Infidex176V-IDENTIDEM.design-remix-counter-train (Autodesk Fusion 360 design; units mm, degrees)
part number: 2026-09-16-11-02-38-314
part number: 2026-09-22-22-56-15-265
part number: 2026-09-22-22-56-15-756
part number: 2026-09-22-22-56-18-900
part number: 2026-09-22-22-56-23-574
part number: 2026-09-22-22-56-29-751
Autodesk Fusion 360 part; units mm, degrees
(part 1 of 7)
ref_plane "WorkPlane1" through (0, 0, 36.8) normal (0, 0, 1) x (1, 0, 0) in component "CT sprocket pinion (tool body)"
sketch "Sketch1" plane through (0, 0, 36.8) normal (0, 0, 1) x (1, 0, 0) in component "CT sprocket pinion (tool body)"
  line L0 (76.2524, -45.6906) -> (76.5417, -45.7362)
  line L1 (76.5417, -45.7362) -> (76.6223, -45.737)
  line L2 (76.6223, -45.737) -> (76.7043, -45.7279)
  line L3 (76.7043, -45.7279) -> (76.7872, -45.7118)
  line L4 (76.7872, -45.7118) -> (76.8707, -45.6898)
  line L5 (76.8707, -45.6898) -> (76.9545, -45.6623)
  line L6 (76.9545, -45.6623) -> (77.0386, -45.6298)
  line L7 (77.0386, -45.6298) -> (77.1226, -45.5924)
  line L8 (77.1226, -45.5924) -> (77.2065, -45.5504)
  line L9 (77.2065, -45.5504) -> (77.2902, -45.5039)
  line L10 (77.2902, -45.5039) -> (77.3734, -45.4529)
  line L11 (77.3734, -45.4529) -> (77.4561, -45.3975)
  line L12 (77.4561, -45.3975) -> (77.5381, -45.3379)
  line L13 (77.5381, -45.3379) -> (77.5398, -45.2526)
  line L14 (77.5398, -45.2526) -> (77.5398, -45.1674)
  line L15 (77.5398, -45.1674) -> (77.5381, -45.0821)
  line L16 (77.5381, -45.0821) -> (77.4561, -45.0225)
  line L17 (77.4561, -45.0225) -> (77.3734, -44.9671)
  line L18 (77.3734, -44.9671) -> (77.2902, -44.9161)
  line L19 (77.2902, -44.9161) -> (77.2065, -44.8696)
  line L20 (77.2065, -44.8696) -> (77.1226, -44.8276)
  line L21 (77.1226, -44.8276) -> (77.0386, -44.7902)
  line L22 (77.0386, -44.7902) -> (76.9545, -44.7577)
  line L23 (76.9545, -44.7577) -> (76.8707, -44.7302)
  line L24 (76.8707, -44.7302) -> (76.7872, -44.7082)
  line L25 (76.7872, -44.7082) -> (76.7043, -44.6921)
  line L26 (76.7043, -44.6921) -> (76.6223, -44.683)
  line L27 (76.6223, -44.683) -> (76.5417, -44.6838)
  line L28 (76.5417, -44.6838) -> (76.2524, -44.7294)
  line L29 (76.2524, -44.7294) -> (76.2228, -44.5689)
  line L30 (76.2228, -44.5689) -> (76.1847, -44.4102)
  line L31 (76.1847, -44.4102) -> (76.1383, -44.2538)
  line L32 (76.1383, -44.2538) -> (76.0838, -44.1)
  line L33 (76.0838, -44.1) -> (76.3571, -43.9948)
  line L34 (76.3571, -43.9948) -> (76.4273, -43.9553)
  line L35 (76.4273, -43.9553) -> (76.4938, -43.9063)
  line L36 (76.4938, -43.9063) -> (76.5575, -43.851)
  line L37 (76.5575, -43.851) -> (76.6188, -43.7901)
  line L38 (76.6188, -43.7901) -> (76.6777, -43.7244)
  line L39 (76.6777, -43.7244) -> (76.7342, -43.6543)
  line L40 (76.7342, -43.6543) -> (76.7883, -43.5799)
  line L41 (76.7883, -43.5799) -> (76.84, -43.5016)
  line L42 (76.84, -43.5016) -> (76.8891, -43.4194)
  line L43 (76.8891, -43.4194) -> (76.9357, -43.3336)
  line L44 (76.9357, -43.3336) -> (76.9797, -43.2444)
  line L45 (76.9797, -43.2444) -> (77.0209, -43.1517)
  line L46 (77.0209, -43.1517) -> (76.9797, -43.077)
  line L47 (76.9797, -43.077) -> (76.937, -43.0032)
  line L48 (76.937, -43.0032) -> (76.893, -42.9302)
  line L49 (76.893, -42.9302) -> (76.7921, -42.9195)
  line L50 (76.7921, -42.9195) -> (76.6929, -42.913)
  line L51 (76.6929, -42.913) -> (76.5953, -42.9104)
  line L52 (76.5953, -42.9104) -> (76.4995, -42.9119)
  line L53 (76.4995, -42.9119) -> (76.4059, -42.9175)
  line L54 (76.4059, -42.9175) -> (76.3144, -42.9272)
  line L55 (76.3144, -42.9272) -> (76.2254, -42.941)
  line L56 (76.2254, -42.941) -> (76.139, -42.9592)
  line L57 (76.139, -42.9592) -> (76.0557, -42.9818)
  line L58 (76.0557, -42.9818) -> (75.9759, -43.0093)
  line L59 (75.9759, -43.0093) -> (75.9003, -43.0424)
  line L60 (75.9003, -43.0424) -> (75.8309, -43.0834)
  line L61 (75.8309, -43.0834) -> (75.6031, -43.2676)
  line L62 (75.6031, -43.2676) -> (75.4972, -43.1434)
  line L63 (75.4972, -43.1434) -> (75.385, -43.025)
  line L64 (75.385, -43.025) -> (75.2666, -42.9128)
  line L65 (75.2666, -42.9128) -> (75.1424, -42.8069)
  line L66 (75.1424, -42.8069) -> (75.3266, -42.5791)
  line L67 (75.3266, -42.5791) -> (75.3676, -42.5097)
  line L68 (75.3676, -42.5097) -> (75.4007, -42.4341)
  line L69 (75.4007, -42.4341) -> (75.4282, -42.3543)
  line L70 (75.4282, -42.3543) -> (75.4508, -42.271)
  line L71 (75.4508, -42.271) -> (75.469, -42.1846)
  line L72 (75.469, -42.1846) -> (75.4828, -42.0956)
  line L73 (75.4828, -42.0956) -> (75.4925, -42.0041)
  line L74 (75.4925, -42.0041) -> (75.4981, -41.9105)
  line L75 (75.4981, -41.9105) -> (75.4996, -41.8147)
  line L76 (75.4996, -41.8147) -> (75.497, -41.7171)
  line L77 (75.497, -41.7171) -> (75.4905, -41.6179)
  line L78 (75.4905, -41.6179) -> (75.4798, -41.517)
  line L79 (75.4798, -41.517) -> (75.4068, -41.473)
  line L80 (75.4068, -41.473) -> (75.333, -41.4303)
  line L81 (75.333, -41.4303) -> (75.2583, -41.3891)
  line L82 (75.2583, -41.3891) -> (75.1656, -41.4303)
  line L83 (75.1656, -41.4303) -> (75.0764, -41.4743)
  line L84 (75.0764, -41.4743) -> (74.9906, -41.5209)
  line L85 (74.9906, -41.5209) -> (74.9084, -41.57)
  line L86 (74.9084, -41.57) -> (74.8301, -41.6217)
  line L87 (74.8301, -41.6217) -> (74.7557, -41.6758)
  line L88 (74.7557, -41.6758) -> (74.6856, -41.7323)
  line L89 (74.6856, -41.7323) -> (74.6199, -41.7912)
  line L90 (74.6199, -41.7912) -> (74.559, -41.8525)
  line L91 (74.559, -41.8525) -> (74.5037, -41.9162)
  line L92 (74.5037, -41.9162) -> (74.4547, -41.9827)
  line L93 (74.4547, -41.9827) -> (74.4152, -42.0529)
  line L94 (74.4152, -42.0529) -> (74.31, -42.3262)
  line L95 (74.31, -42.3262) -> (74.1562, -42.2717)
  line L96 (74.1562, -42.2717) -> (73.9998, -42.2253)
  line L97 (73.9998, -42.2253) -> (73.8411, -42.1872)
  line L98 (73.8411, -42.1872) -> (73.6806, -42.1576)
  line L99 (73.6806, -42.1576) -> (73.7262, -41.8683)
  line L100 (73.7262, -41.8683) -> (73.727, -41.7877)
  line L101 (73.727, -41.7877) -> (73.7179, -41.7057)
  line L102 (73.7179, -41.7057) -> (73.7018, -41.6228)
  line L103 (73.7018, -41.6228) -> (73.6798, -41.5393)
  line L104 (73.6798, -41.5393) -> (73.6523, -41.4555)
  line L105 (73.6523, -41.4555) -> (73.6198, -41.3714)
  line L106 (73.6198, -41.3714) -> (73.5824, -41.2874)
  line L107 (73.5824, -41.2874) -> (73.5404, -41.2035)
  line L108 (73.5404, -41.2035) -> (73.4939, -41.1198)
  line L109 (73.4939, -41.1198) -> (73.4429, -41.0366)
  line L110 (73.4429, -41.0366) -> (73.3875, -40.9539)
  line L111 (73.3875, -40.9539) -> (73.3279, -40.8719)
  line L112 (73.3279, -40.8719) -> (73.2426, -40.8702)
  line L113 (73.2426, -40.8702) -> (73.1574, -40.8702)
  line L114 (73.1574, -40.8702) -> (73.0721, -40.8719)
  line L115 (73.0721, -40.8719) -> (73.0125, -40.9539)
  line L116 (73.0125, -40.9539) -> (72.9571, -41.0366)
  line L117 (72.9571, -41.0366) -> (72.9061, -41.1198)
  line L118 (72.9061, -41.1198) -> (72.8596, -41.2035)
  line L119 (72.8596, -41.2035) -> (72.8176, -41.2874)
  line L120 (72.8176, -41.2874) -> (72.7802, -41.3714)
  line L121 (72.7802, -41.3714) -> (72.7477, -41.4555)
  line L122 (72.7477, -41.4555) -> (72.7202, -41.5393)
  line L123 (72.7202, -41.5393) -> (72.6982, -41.6228)
  line L124 (72.6982, -41.6228) -> (72.6821, -41.7057)
  line L125 (72.6821, -41.7057) -> (72.673, -41.7877)
  line L126 (72.673, -41.7877) -> (72.6738, -41.8683)
  line L127 (72.6738, -41.8683) -> (72.7194, -42.1576)
  line L128 (72.7194, -42.1576) -> (72.5589, -42.1872)
  line L129 (72.5589, -42.1872) -> (72.4002, -42.2253)
  line L130 (72.4002, -42.2253) -> (72.2438, -42.2717)
  line L131 (72.2438, -42.2717) -> (72.09, -42.3262)
  line L132 (72.09, -42.3262) -> (71.9848, -42.0529)
  line L133 (71.9848, -42.0529) -> (71.9453, -41.9827)
  line L134 (71.9453, -41.9827) -> (71.8963, -41.9162)
  line L135 (71.8963, -41.9162) -> (71.841, -41.8525)
  line L136 (71.841, -41.8525) -> (71.7801, -41.7912)
  line L137 (71.7801, -41.7912) -> (71.7144, -41.7323)
  line L138 (71.7144, -41.7323) -> (71.6443, -41.6758)
  line L139 (71.6443, -41.6758) -> (71.5699, -41.6217)
  line L140 (71.5699, -41.6217) -> (71.4916, -41.57)
  line L141 (71.4916, -41.57) -> (71.4094, -41.5209)
  line L142 (71.4094, -41.5209) -> (71.3236, -41.4743)
  line L143 (71.3236, -41.4743) -> (71.2344, -41.4303)
  line L144 (71.2344, -41.4303) -> (71.1417, -41.3891)
  line L145 (71.1417, -41.3891) -> (71.067, -41.4303)
  line L146 (71.067, -41.4303) -> (70.9932, -41.473)
  line L147 (70.9932, -41.473) -> (70.9202, -41.517)
  line L148 (70.9202, -41.517) -> (70.9095, -41.6179)
  line L149 (70.9095, -41.6179) -> (70.903, -41.7171)
  line L150 (70.903, -41.7171) -> (70.9004, -41.8147)
  line L151 (70.9004, -41.8147) -> (70.9019, -41.9105)
  line L152 (70.9019, -41.9105) -> (70.9075, -42.0041)
  line L153 (70.9075, -42.0041) -> (70.9172, -42.0956)
  line L154 (70.9172, -42.0956) -> (70.931, -42.1846)
  line L155 (70.931, -42.1846) -> (70.9492, -42.271)
  line L156 (70.9492, -42.271) -> (70.9718, -42.3543)
  line L157 (70.9718, -42.3543) -> (70.9993, -42.4341)
  line L158 (70.9993, -42.4341) -> (71.0324, -42.5097)
  line L159 (71.0324, -42.5097) -> (71.0734, -42.5791)
  line L160 (71.0734, -42.5791) -> (71.2576, -42.8069)
  line L161 (71.2576, -42.8069) -> (71.1334, -42.9128)
  line L162 (71.1334, -42.9128) -> (71.015, -43.025)
  line L163 (71.015, -43.025) -> (70.9028, -43.1434)
  line L164 (70.9028, -43.1434) -> (70.7969, -43.2676)
  line L165 (70.7969, -43.2676) -> (70.5691, -43.0834)
  line L166 (70.5691, -43.0834) -> (70.4997, -43.0424)
  line L167 (70.4997, -43.0424) -> (70.4241, -43.0093)
  line L168 (70.4241, -43.0093) -> (70.3443, -42.9818)
  line L169 (70.3443, -42.9818) -> (70.261, -42.9592)
  line L170 (70.261, -42.9592) -> (70.1746, -42.941)
  line L171 (70.1746, -42.941) -> (70.0856, -42.9272)
  line L172 (70.0856, -42.9272) -> (69.9941, -42.9175)
  line L173 (69.9941, -42.9175) -> (69.9005, -42.9119)
  line L174 (69.9005, -42.9119) -> (69.8047, -42.9104)
  line L175 (69.8047, -42.9104) -> (69.7071, -42.913)
  line L176 (69.7071, -42.913) -> (69.6079, -42.9195)
  line L177 (69.6079, -42.9195) -> (69.507, -42.9302)
  line L178 (69.507, -42.9302) -> (69.463, -43.0032)
  line L179 (69.463, -43.0032) -> (69.4203, -43.077)
  line L180 (69.4203, -43.077) -> (69.3791, -43.1517)
  line L181 (69.3791, -43.1517) -> (69.4203, -43.2444)
  line L182 (69.4203, -43.2444) -> (69.4643, -43.3336)
  line L183 (69.4643, -43.3336) -> (69.5109, -43.4194)
  line L184 (69.5109, -43.4194) -> (69.56, -43.5016)
  line L185 (69.56, -43.5016) -> (69.6117, -43.5799)
  line L186 (69.6117, -43.5799) -> (69.6658, -43.6543)
  line L187 (69.6658, -43.6543) -> (69.7223, -43.7244)
  line L188 (69.7223, -43.7244) -> (69.7812, -43.7901)
  line L189 (69.7812, -43.7901) -> (69.8425, -43.851)
  line L190 (69.8425, -43.851) -> (69.9062, -43.9063)
  line L191 (69.9062, -43.9063) -> (69.9727, -43.9553)
  line L192 (69.9727, -43.9553) -> (70.0429, -43.9948)
  line L193 (70.0429, -43.9948) -> (70.3162, -44.1)
  line L194 (70.3162, -44.1) -> (70.2617, -44.2538)
  line L195 (70.2617, -44.2538) -> (70.2153, -44.4102)
  line L196 (70.2153, -44.4102) -> (70.1772, -44.5689)
  line L197 (70.1772, -44.5689) -> (70.1476, -44.7294)
  line L198 (70.1476, -44.7294) -> (69.8583, -44.6838)
  line L199 (69.8583, -44.6838) -> (69.7777, -44.683)
  line L200 (69.7777, -44.683) -> (69.6957, -44.6921)
  line L201 (69.6957, -44.6921) -> (69.6128, -44.7082)
  line L202 (69.6128, -44.7082) -> (69.5293, -44.7302)
  line L203 (69.5293, -44.7302) -> (69.4455, -44.7577)
  line L204 (69.4455, -44.7577) -> (69.3614, -44.7902)
  line L205 (69.3614, -44.7902) -> (69.2774, -44.8276)
  line L206 (69.2774, -44.8276) -> (69.1935, -44.8696)
  line L207 (69.1935, -44.8696) -> (69.1098, -44.9161)
  line L208 (69.1098, -44.9161) -> (69.0266, -44.9671)
  line L209 (69.0266, -44.9671) -> (68.9439, -45.0225)
  line L210 (68.9439, -45.0225) -> (68.8619, -45.0821)
  line L211 (68.8619, -45.0821) -> (68.8602, -45.1674)
  line L212 (68.8602, -45.1674) -> (68.8602, -45.2526)
  line L213 (68.8602, -45.2526) -> (68.8619, -45.3379)
  line L214 (68.8619, -45.3379) -> (68.9439, -45.3975)
  line L215 (68.9439, -45.3975) -> (69.0266, -45.4529)
  line L216 (69.0266, -45.4529) -> (69.1098, -45.5039)
  line L217 (69.1098, -45.5039) -> (69.1935, -45.5504)
  line L218 (69.1935, -45.5504) -> (69.2774, -45.5924)
  line L219 (69.2774, -45.5924) -> (69.3614, -45.6298)
  line L220 (69.3614, -45.6298) -> (69.4455, -45.6623)
  line L221 (69.4455, -45.6623) -> (69.5293, -45.6898)
  line L222 (69.5293, -45.6898) -> (69.6128, -45.7118)
  line L223 (69.6128, -45.7118) -> (69.6957, -45.7279)
  line L224 (69.6957, -45.7279) -> (69.7777, -45.737)
  line L225 (69.7777, -45.737) -> (69.8583, -45.7362)
  line L226 (69.8583, -45.7362) -> (70.1476, -45.6906)
  line L227 (70.1476, -45.6906) -> (70.1772, -45.8511)
  line L228 (70.1772, -45.8511) -> (70.2153, -46.0098)
  line L229 (70.2153, -46.0098) -> (70.2617, -46.1662)
  line L230 (70.2617, -46.1662) -> (70.3162, -46.32)
  line L231 (70.3162, -46.32) -> (70.0429, -46.4252)
  line L232 (70.0429, -46.4252) -> (69.9727, -46.4647)
  line L233 (69.9727, -46.4647) -> (69.9062, -46.5137)
  line L234 (69.9062, -46.5137) -> (69.8425, -46.569)
  line L235 (69.8425, -46.569) -> (69.7812, -46.6299)
  line L236 (69.7812, -46.6299) -> (69.7223, -46.6956)
  line L237 (69.7223, -46.6956) -> (69.6658, -46.7657)
  line L238 (69.6658, -46.7657) -> (69.6117, -46.8401)
  line L239 (69.6117, -46.8401) -> (69.56, -46.9184)
  line L240 (69.56, -46.9184) -> (69.5109, -47.0006)
  line L241 (69.5109, -47.0006) -> (69.4643, -47.0864)
  line L242 (69.4643, -47.0864) -> (69.4203, -47.1756)
  line L243 (69.4203, -47.1756) -> (69.3791, -47.2683)
  line L244 (69.3791, -47.2683) -> (69.4203, -47.343)
  line L245 (69.4203, -47.343) -> (69.463, -47.4168)
  line L246 (69.463, -47.4168) -> (69.507, -47.4898)
  line L247 (69.507, -47.4898) -> (69.6079, -47.5005)
  line L248 (69.6079, -47.5005) -> (69.7071, -47.507)
  line L249 (69.7071, -47.507) -> (69.8047, -47.5096)
  line L250 (69.8047, -47.5096) -> (69.9005, -47.5081)
  line L251 (69.9005, -47.5081) -> (69.9941, -47.5025)
  line L252 (69.9941, -47.5025) -> (70.0856, -47.4928)
  line L253 (70.0856, -47.4928) -> (70.1746, -47.479)
  line L254 (70.1746, -47.479) -> (70.261, -47.4608)
  line L255 (70.261, -47.4608) -> (70.3443, -47.4382)
  line L256 (70.3443, -47.4382) -> (70.4241, -47.4107)
  line L257 (70.4241, -47.4107) -> (70.4997, -47.3776)
  line L258 (70.4997, -47.3776) -> (70.5691, -47.3366)
  line L259 (70.5691, -47.3366) -> (70.7969, -47.1524)
  line L260 (70.7969, -47.1524) -> (70.9028, -47.2766)
  line L261 (70.9028, -47.2766) -> (71.015, -47.395)
  line L262 (71.015, -47.395) -> (71.1334, -47.5072)
  line L263 (71.1334, -47.5072) -> (71.2576, -47.6131)
  line L264 (71.2576, -47.6131) -> (71.0734, -47.8409)
  line L265 (71.0734, -47.8409) -> (71.0324, -47.9103)
  line L266 (71.0324, -47.9103) -> (70.9993, -47.9859)
  line L267 (70.9993, -47.9859) -> (70.9718, -48.0657)
  line L268 (70.9718, -48.0657) -> (70.9492, -48.149)
  line L269 (70.9492, -48.149) -> (70.931, -48.2354)
  line L270 (70.931, -48.2354) -> (70.9172, -48.3244)
  line L271 (70.9172, -48.3244) -> (70.9075, -48.4159)
  line L272 (70.9075, -48.4159) -> (70.9019, -48.5095)
  line L273 (70.9019, -48.5095) -> (70.9004, -48.6053)
  line L274 (70.9004, -48.6053) -> (70.903, -48.7029)
  line L275 (70.903, -48.7029) -> (70.9095, -48.8021)
  line L276 (70.9095, -48.8021) -> (70.9202, -48.903)
  line L277 (70.9202, -48.903) -> (70.9932, -48.947)
  line L278 (70.9932, -48.947) -> (71.067, -48.9897)
  line L279 (71.067, -48.9897) -> (71.1417, -49.0309)
  line L280 (71.1417, -49.0309) -> (71.2344, -48.9897)
  line L281 (71.2344, -48.9897) -> (71.3236, -48.9457)
  line L282 (71.3236, -48.9457) -> (71.4094, -48.8991)
  line L283 (71.4094, -48.8991) -> (71.4916, -48.85)
  line L284 (71.4916, -48.85) -> (71.5699, -48.7983)
  line L285 (71.5699, -48.7983) -> (71.6443, -48.7442)
  line L286 (71.6443, -48.7442) -> (71.7144, -48.6877)
  line L287 (71.7144, -48.6877) -> (71.7801, -48.6288)
  line L288 (71.7801, -48.6288) -> (71.841, -48.5675)
  line L289 (71.841, -48.5675) -> (71.8963, -48.5038)
  line L290 (71.8963, -48.5038) -> (71.9453, -48.4373)
  line L291 (71.9453, -48.4373) -> (71.9848, -48.3671)
  line L292 (71.9848, -48.3671) -> (72.09, -48.0938)
  line L293 (72.09, -48.0938) -> (72.2438, -48.1483)
  line L294 (72.2438, -48.1483) -> (72.4002, -48.1947)
  line L295 (72.4002, -48.1947) -> (72.5589, -48.2328)
  line L296 (72.5589, -48.2328) -> (72.7194, -48.2624)
  line L297 (72.7194, -48.2624) -> (72.6738, -48.5517)
  line L298 (72.6738, -48.5517) -> (72.673, -48.6323)
  line L299 (72.673, -48.6323) -> (72.6821, -48.7143)
  line L300 (72.6821, -48.7143) -> (72.6982, -48.7972)
  line L301 (72.6982, -48.7972) -> (72.7202, -48.8807)
  line L302 (72.7202, -48.8807) -> (72.7477, -48.9645)
  line L303 (72.7477, -48.9645) -> (72.7802, -49.0486)
  line L304 (72.7802, -49.0486) -> (72.8176, -49.1326)
  line L305 (72.8176, -49.1326) -> (72.8596, -49.2165)
  line L306 (72.8596, -49.2165) -> (72.9061, -49.3002)
  line L307 (72.9061, -49.3002) -> (72.9571, -49.3834)
  line L308 (72.9571, -49.3834) -> (73.0125, -49.4661)
  line L309 (73.0125, -49.4661) -> (73.0721, -49.5481)
  line L310 (73.0721, -49.5481) -> (73.1574, -49.5498)
  line L311 (73.1574, -49.5498) -> (73.2426, -49.5498)
  line L312 (73.2426, -49.5498) -> (73.3279, -49.5481)
  line L313 (73.3279, -49.5481) -> (73.3875, -49.4661)
  line L314 (73.3875, -49.4661) -> (73.4429, -49.3834)
  line L315 (73.4429, -49.3834) -> (73.4939, -49.3002)
  line L316 (73.4939, -49.3002) -> (73.5404, -49.2165)
  line L317 (73.5404, -49.2165) -> (73.5824, -49.1326)
  line L318 (73.5824, -49.1326) -> (73.6198, -49.0486)
  line L319 (73.6198, -49.0486) -> (73.6523, -48.9645)
  line L320 (73.6523, -48.9645) -> (73.6798, -48.8807)
  line L321 (73.6798, -48.8807) -> (73.7018, -48.7972)
  line L322 (73.7018, -48.7972) -> (73.7179, -48.7143)
  line L323 (73.7179, -48.7143) -> (73.727, -48.6323)
  line L324 (73.727, -48.6323) -> (73.7262, -48.5517)
  line L325 (73.7262, -48.5517) -> (73.6806, -48.2624)
  line L326 (73.6806, -48.2624) -> (73.8411, -48.2328)
  line L327 (73.8411, -48.2328) -> (73.9998, -48.1947)
  line L328 (73.9998, -48.1947) -> (74.1562, -48.1483)
  line L329 (74.1562, -48.1483) -> (74.31, -48.0938)
  line L330 (74.31, -48.0938) -> (74.4152, -48.3671)
  line L331 (74.4152, -48.3671) -> (74.4547, -48.4373)
  line L332 (74.4547, -48.4373) -> (74.5037, -48.5038)
  line L333 (74.5037, -48.5038) -> (74.559, -48.5675)
  line L334 (74.559, -48.5675) -> (74.6199, -48.6288)
  line L335 (74.6199, -48.6288) -> (74.6856, -48.6877)
  line L336 (74.6856, -48.6877) -> (74.7557, -48.7442)
  line L337 (74.7557, -48.7442) -> (74.8301, -48.7983)
  line L338 (74.8301, -48.7983) -> (74.9084, -48.85)
  line L339 (74.9084, -48.85) -> (74.9906, -48.8991)
  line L340 (74.9906, -48.8991) -> (75.0764, -48.9457)
  line L341 (75.0764, -48.9457) -> (75.1656, -48.9897)
  line L342 (75.1656, -48.9897) -> (75.2583, -49.0309)
  line L343 (75.2583, -49.0309) -> (75.333, -48.9897)
  line L344 (75.333, -48.9897) -> (75.4068, -48.947)
  line L345 (75.4068, -48.947) -> (75.4798, -48.903)
  line L346 (75.4798, -48.903) -> (75.4905, -48.8021)
  line L347 (75.4905, -48.8021) -> (75.497, -48.7029)
  line L348 (75.497, -48.7029) -> (75.4996, -48.6053)
  line L349 (75.4996, -48.6053) -> (75.4981, -48.5095)
  line L350 (75.4981, -48.5095) -> (75.4925, -48.4159)
  line L351 (75.4925, -48.4159) -> (75.4828, -48.3244)
  line L352 (75.4828, -48.3244) -> (75.469, -48.2354)
  line L353 (75.469, -48.2354) -> (75.4508, -48.149)
  line L354 (75.4508, -48.149) -> (75.4282, -48.0657)
  line L355 (75.4282, -48.0657) -> (75.4007, -47.9859)
  line L356 (75.4007, -47.9859) -> (75.3676, -47.9103)
  line L357 (75.3676, -47.9103) -> (75.3266, -47.8409)
  line L358 (75.3266, -47.8409) -> (75.1424, -47.6131)
  line L359 (75.1424, -47.6131) -> (75.2666, -47.5072)
  line L360 (75.2666, -47.5072) -> (75.385, -47.395)
  line L361 (75.385, -47.395) -> (75.4972, -47.2766)
  line L362 (75.4972, -47.2766) -> (75.6031, -47.1524)
  line L363 (75.6031, -47.1524) -> (75.8309, -47.3366)
  line L364 (75.8309, -47.3366) -> (75.9003, -47.3776)
  line L365 (75.9003, -47.3776) -> (75.9759, -47.4107)
  line L366 (75.9759, -47.4107) -> (76.0557, -47.4382)
  line L367 (76.0557, -47.4382) -> (76.139, -47.4608)
  line L368 (76.139, -47.4608) -> (76.2254, -47.479)
  line L369 (76.2254, -47.479) -> (76.3144, -47.4928)
  line L370 (76.3144, -47.4928) -> (76.4059, -47.5025)
  line L371 (76.4059, -47.5025) -> (76.4995, -47.5081)
  line L372 (76.4995, -47.5081) -> (76.5953, -47.5096)
  line L373 (76.5953, -47.5096) -> (76.6929, -47.507)
  line L374 (76.6929, -47.507) -> (76.7921, -47.5005)
  line L375 (76.7921, -47.5005) -> (76.893, -47.4898)
  line L376 (76.893, -47.4898) -> (76.937, -47.4168)
  line L377 (76.937, -47.4168) -> (76.9797, -47.343)
  line L378 (76.9797, -47.343) -> (77.0209, -47.2683)
  line L379 (77.0209, -47.2683) -> (76.9797, -47.1756)
  line L380 (76.9797, -47.1756) -> (76.9357, -47.0864)
  line L381 (76.9357, -47.0864) -> (76.8891, -47.0006)
  line L382 (76.8891, -47.0006) -> (76.84, -46.9184)
  line L383 (76.84, -46.9184) -> (76.7883, -46.8401)
  line L384 (76.7883, -46.8401) -> (76.7342, -46.7657)
  line L385 (76.7342, -46.7657) -> (76.6777, -46.6956)
  line L386 (76.6777, -46.6956) -> (76.6188, -46.6299)
  line L387 (76.6188, -46.6299) -> (76.5575, -46.569)
  line L388 (76.5575, -46.569) -> (76.4938, -46.5137)
  line L389 (76.4938, -46.5137) -> (76.4273, -46.4647)
  line L390 (76.4273, -46.4647) -> (76.3571, -46.4252)
  line L391 (76.3571, -46.4252) -> (76.0838, -46.32)
  line L392 (76.0838, -46.32) -> (76.1383, -46.1662)
  line L393 (76.1383, -46.1662) -> (76.1847, -46.0098)
  line L394 (76.1847, -46.0098) -> (76.2228, -45.8511)
  line L395 (76.2228, -45.8511) -> (76.2524, -45.6906)
extrude "Extrude1" add sketch "Sketch1" along normal blind 2 makes body 1 in component "CT sprocket pinion (tool body)"
ref_plane "WorkPlane1" through (0, 0, 36.8) normal (0, 0, 1) x (1, 0, 0) in component "CT idler 1"
sketch "Sketch1 (2)" plane through (0, 0, 36.8) normal (0, 0, 1) x (1, 0, 0) in component "CT idler 1"
  line L0 (81.6289, -58.8365) -> (82.0394, -58.8569)
  line L1 (82.0394, -58.8569) -> (82.1146, -58.8542)
  line L2 (82.1146, -58.8542) -> (82.19, -58.846)
  line L3 (82.19, -58.846) -> (82.2655, -58.8342)
  line L4 (82.2655, -58.8342) -> (82.3412, -58.8194)
  line L5 (82.3412, -58.8194) -> (82.4169, -58.802)
  line L6 (82.4169, -58.802) -> (82.4927, -58.7822)
  line L7 (82.4927, -58.7822) -> (82.5685, -58.7601)
  line L8 (82.5685, -58.7601) -> (82.6443, -58.7359)
  line L9 (82.6443, -58.7359) -> (82.7201, -58.7098)
  line L10 (82.7201, -58.7098) -> (82.7959, -58.6817)
  line L11 (82.7959, -58.6817) -> (82.8716, -58.6517)
  line L12 (82.8716, -58.6517) -> (82.9473, -58.6199)
  line L13 (82.9473, -58.6199) -> (82.9493, -58.4792)
  line L14 (82.9493, -58.4792) -> (82.9493, -58.3386)
  line L15 (82.9493, -58.3386) -> (82.9473, -58.1979)
  line L16 (82.9473, -58.1979) -> (82.8716, -58.1661)
  line L17 (82.8716, -58.1661) -> (82.7959, -58.1361)
  line L18 (82.7959, -58.1361) -> (82.7201, -58.108)
  line L19 (82.7201, -58.108) -> (82.6443, -58.0818)
  line L20 (82.6443, -58.0818) -> (82.5685, -58.0577)
  line L21 (82.5685, -58.0577) -> (82.4927, -58.0356)
  line L22 (82.4927, -58.0356) -> (82.4169, -58.0158)
  line L23 (82.4169, -58.0158) -> (82.3412, -57.9984)
  line L24 (82.3412, -57.9984) -> (82.2655, -57.9836)
  line L25 (82.2655, -57.9836) -> (82.19, -57.9718)
  line L26 (82.19, -57.9718) -> (82.1146, -57.9636)
  line L27 (82.1146, -57.9636) -> (82.0394, -57.9609)
  line L28 (82.0394, -57.9609) -> (81.6289, -57.9813)
  line L29 (81.6289, -57.9813) -> (81.616, -57.7729)
  line L30 (81.616, -57.7729) -> (81.5981, -57.565)
  line L31 (81.5981, -57.565) -> (81.5751, -57.3575)
  line L32 (81.5751, -57.3575) -> (81.5471, -57.1506)
  line L33 (81.5471, -57.1506) -> (81.9537, -57.0906)
  line L34 (81.9537, -57.0906) -> (82.0269, -57.0732)
  line L35 (82.0269, -57.0732) -> (82.0992, -57.0505)
  line L36 (82.0992, -57.0505) -> (82.171, -57.0242)
  line L37 (82.171, -57.0242) -> (82.2423, -56.9949)
  line L38 (82.2423, -56.9949) -> (82.3132, -56.9631)
  line L39 (82.3132, -56.9631) -> (82.3837, -56.9288)
  line L40 (82.3837, -56.9288) -> (82.4537, -56.8924)
  line L41 (82.4537, -56.8924) -> (82.5234, -56.8539)
  line L42 (82.5234, -56.8539) -> (82.5926, -56.8134)
  line L43 (82.5926, -56.8134) -> (82.6614, -56.7711)
  line L44 (82.6614, -56.7711) -> (82.7299, -56.7269)
  line L45 (82.7299, -56.7269) -> (82.7979, -56.681)
  line L46 (82.7979, -56.681) -> (82.7724, -56.5426)
  line L47 (82.7724, -56.5426) -> (82.7449, -56.4047)
  line L48 (82.7449, -56.4047) -> (82.7155, -56.2671)
  line L49 (82.7155, -56.2671) -> (82.6351, -56.2507)
  line L50 (82.6351, -56.2507) -> (82.555, -56.2361)
  line L51 (82.555, -56.2361) -> (82.4752, -56.2233)
  line L52 (82.4752, -56.2233) -> (82.3958, -56.2124)
  line L53 (82.3958, -56.2124) -> (82.3167, -56.2035)
  line L54 (82.3167, -56.2035) -> (82.238, -56.1966)
  line L55 (82.238, -56.1966) -> (82.1598, -56.192)
  line L56 (82.1598, -56.192) -> (82.0822, -56.1896)
  line L57 (82.0822, -56.1896) -> (82.0051, -56.1899)
  line L58 (82.0051, -56.1899) -> (81.9287, -56.1931)
  line L59 (81.9287, -56.1931) -> (81.8531, -56.1998)
  line L60 (81.8531, -56.1998) -> (81.7789, -56.2117)
  line L61 (81.7789, -56.2117) -> (81.3802, -56.3119)
  line L62 (81.3802, -56.3119) -> (81.3269, -56.11)
  line L63 (81.3269, -56.11) -> (81.2688, -55.9095)
  line L64 (81.2688, -55.9095) -> (81.2058, -55.7105)
  line L65 (81.2058, -55.7105) -> (81.1379, -55.5131)
  line L66 (81.1379, -55.5131) -> (81.525, -55.3749)
  line L67 (81.525, -55.3749) -> (81.5934, -55.3436)
  line L68 (81.5934, -55.3436) -> (81.6599, -55.3072)
  line L69 (81.6599, -55.3072) -> (81.7252, -55.2674)
  line L70 (81.7252, -55.2674) -> (81.7895, -55.2248)
  line L71 (81.7895, -55.2248) -> (81.8528, -55.1797)
  line L72 (81.8528, -55.1797) -> (81.9152, -55.1324)
  line L73 (81.9152, -55.1324) -> (81.9768, -55.083)
  line L74 (81.9768, -55.083) -> (82.0376, -55.0316)
  line L75 (82.0376, -55.0316) -> (82.0976, -54.9784)
  line L76 (82.0976, -54.9784) -> (82.1568, -54.9235)
  line L77 (82.1568, -54.9235) -> (82.2153, -54.8668)
  line L78 (82.2153, -54.8668) -> (82.2731, -54.8085)
  line L79 (82.2731, -54.8085) -> (82.2211, -54.6778)
  line L80 (82.2211, -54.6778) -> (82.1673, -54.5478)
  line L81 (82.1673, -54.5478) -> (82.1116, -54.4186)
  line L82 (82.1116, -54.4186) -> (82.0295, -54.4182)
  line L83 (82.0295, -54.4182) -> (81.9481, -54.4195)
  line L84 (81.9481, -54.4195) -> (81.8673, -54.4225)
  line L85 (81.8673, -54.4225) -> (81.7873, -54.4273)
  line L86 (81.7873, -54.4273) -> (81.708, -54.434)
  line L87 (81.708, -54.434) -> (81.6295, -54.4426)
  line L88 (81.6295, -54.4426) -> (81.5519, -54.4533)
  line L89 (81.5519, -54.4533) -> (81.4753, -54.4662)
  line L90 (81.4753, -54.4662) -> (81.3997, -54.4815)
  line L91 (81.3997, -54.4815) -> (81.3254, -54.4995)
  line L92 (81.3254, -54.4995) -> (81.2526, -54.5208)
  line L93 (81.2526, -54.5208) -> (81.1821, -54.547)
  line L94 (81.1821, -54.547) -> (80.8107, -54.723)
  line L95 (80.8107, -54.723) -> (80.719, -54.5355)
  line L96 (80.719, -54.5355) -> (80.6229, -54.3502)
  line L97 (80.6229, -54.3502) -> (80.5222, -54.1673)
  line L98 (80.5222, -54.1673) -> (80.4172, -53.9869)
  line L99 (80.4172, -53.9869) -> (80.7699, -53.7758)
  line L100 (80.7699, -53.7758) -> (80.8309, -53.7318)
  line L101 (80.8309, -53.7318) -> (80.889, -53.6831)
  line L102 (80.889, -53.6831) -> (80.9453, -53.6313)
  line L103 (80.9453, -53.6313) -> (81, -53.577)
  line L104 (81, -53.577) -> (81.0532, -53.5204)
  line L105 (81.0532, -53.5204) -> (81.1052, -53.4618)
  line L106 (81.1052, -53.4618) -> (81.156, -53.4014)
  line L107 (81.156, -53.4014) -> (81.2056, -53.3391)
  line L108 (81.2056, -53.3391) -> (81.2541, -53.2753)
  line L109 (81.2541, -53.2753) -> (81.3015, -53.2098)
  line L110 (81.3015, -53.2098) -> (81.3478, -53.1428)
  line L111 (81.3478, -53.1428) -> (81.3931, -53.0743)
  line L112 (81.3931, -53.0743) -> (81.3166, -52.9563)
  line L113 (81.3166, -52.9563) -> (81.2384, -52.8393)
  line L114 (81.2384, -52.8393) -> (81.1586, -52.7234)
  line L115 (81.1586, -52.7234) -> (81.078, -52.7391)
  line L116 (81.078, -52.7391) -> (80.9984, -52.7562)
  line L117 (80.9984, -52.7562) -> (80.9198, -52.7749)
  line L118 (80.9198, -52.7749) -> (80.8422, -52.7953)
  line L119 (80.8422, -52.7953) -> (80.7658, -52.8173)
  line L120 (80.7658, -52.8173) -> (80.6905, -52.8411)
  line L121 (80.6905, -52.8411) -> (80.6164, -52.8667)
  line L122 (80.6164, -52.8667) -> (80.5438, -52.8943)
  line L123 (80.5438, -52.8943) -> (80.4727, -52.924)
  line L124 (80.4727, -52.924) -> (80.4033, -52.9562)
  line L125 (80.4033, -52.9562) -> (80.3361, -52.9913)
  line L126 (80.3361, -52.9913) -> (80.2721, -53.0307)
  line L127 (80.2721, -53.0307) -> (79.9421, -53.2758)
  line L128 (79.9421, -53.2758) -> (79.8156, -53.1097)
  line L129 (79.8156, -53.1097) -> (79.6851, -52.9468)
  line L130 (79.6851, -52.9468) -> (79.5508, -52.787)
  line L131 (79.5508, -52.787) -> (79.4126, -52.6306)
  line L132 (79.4126, -52.6306) -> (79.7173, -52.3547)
  line L133 (79.7173, -52.3547) -> (79.7685, -52.2997)
  line L134 (79.7685, -52.2997) -> (79.816, -52.2406)
  line L135 (79.816, -52.2406) -> (79.8611, -52.1788)
  line L136 (79.8611, -52.1788) -> (79.9041, -52.1149)
  line L137 (79.9041, -52.1149) -> (79.9454, -52.049)
  line L138 (79.9454, -52.049) -> (79.9849, -51.9814)
  line L139 (79.9849, -51.9814) -> (80.0229, -51.9122)
  line L140 (80.0229, -51.9122) -> (80.0595, -51.8415)
  line L141 (80.0595, -51.8415) -> (80.0945, -51.7694)
  line L142 (80.0945, -51.7694) -> (80.1283, -51.6959)
  line L143 (80.1283, -51.6959) -> (80.1606, -51.6212)
  line L144 (80.1606, -51.6212) -> (80.1916, -51.5452)
  line L145 (80.1916, -51.5452) -> (80.0936, -51.4443)
  line L146 (80.0936, -51.4443) -> (79.9941, -51.3448)
  line L147 (79.9941, -51.3448) -> (79.8932, -51.2468)
  line L148 (79.8932, -51.2468) -> (79.8173, -51.2778)
  line L149 (79.8173, -51.2778) -> (79.7425, -51.3102)
  line L150 (79.7425, -51.3102) -> (79.6691, -51.3439)
  line L151 (79.6691, -51.3439) -> (79.5969, -51.379)
  line L152 (79.5969, -51.379) -> (79.5262, -51.4155)
  line L153 (79.5262, -51.4155) -> (79.457, -51.4535)
  line L154 (79.457, -51.4535) -> (79.3894, -51.493)
  line L155 (79.3894, -51.493) -> (79.3236, -51.5343)
  line L156 (79.3236, -51.5343) -> (79.2596, -51.5773)
  line L157 (79.2596, -51.5773) -> (79.1979, -51.6224)
  line L158 (79.1979, -51.6224) -> (79.1388, -51.6699)
  line L159 (79.1388, -51.6699) -> (79.0837, -51.7211)
  line L160 (79.0837, -51.7211) -> (78.8078, -52.0259)
  line L161 (78.8078, -52.0259) -> (78.6514, -51.8877)
  line L162 (78.6514, -51.8877) -> (78.4916, -51.7533)
  line L163 (78.4916, -51.7533) -> (78.3287, -51.6228)
  line L164 (78.3287, -51.6228) -> (78.1626, -51.4963)
  line L165 (78.1626, -51.4963) -> (78.4077, -51.1663)
  line L166 (78.4077, -51.1663) -> (78.4471, -51.1023)
  line L167 (78.4471, -51.1023) -> (78.4822, -51.0351)
  line L168 (78.4822, -51.0351) -> (78.5144, -50.9657)
  line L169 (78.5144, -50.9657) -> (78.5441, -50.8946)
  line L170 (78.5441, -50.8946) -> (78.5717, -50.822)
  line L171 (78.5717, -50.822) -> (78.5974, -50.748)
  line L172 (78.5974, -50.748) -> (78.6211, -50.6727)
  line L173 (78.6211, -50.6727) -> (78.6431, -50.5962)
  line L174 (78.6431, -50.5962) -> (78.6635, -50.5186)
  line L175 (78.6635, -50.5186) -> (78.6822, -50.44)
  line L176 (78.6822, -50.44) -> (78.6994, -50.3604)
  line L177 (78.6994, -50.3604) -> (78.715, -50.2798)
  line L178 (78.715, -50.2798) -> (78.5991, -50.2)
  line L179 (78.5991, -50.2) -> (78.4822, -50.1219)
  line L180 (78.4822, -50.1219) -> (78.3641, -50.0454)
  line L181 (78.3641, -50.0454) -> (78.2956, -50.0906)
  line L182 (78.2956, -50.0906) -> (78.2286, -50.1369)
  line L183 (78.2286, -50.1369) -> (78.1632, -50.1843)
  line L184 (78.1632, -50.1843) -> (78.0993, -50.2328)
  line L185 (78.0993, -50.2328) -> (78.0371, -50.2824)
  line L186 (78.0371, -50.2824) -> (77.9766, -50.3332)
  line L187 (77.9766, -50.3332) -> (77.918, -50.3852)
  line L188 (77.918, -50.3852) -> (77.8615, -50.4385)
  line L189 (77.8615, -50.4385) -> (77.8071, -50.4932)
  line L190 (77.8071, -50.4932) -> (77.7553, -50.5494)
  line L191 (77.7553, -50.5494) -> (77.7067, -50.6076)
  line L192 (77.7067, -50.6076) -> (77.6626, -50.6685)
  line L193 (77.6626, -50.6685) -> (77.4515, -51.0212)
  line L194 (77.4515, -51.0212) -> (77.2711, -50.9162)
  line L195 (77.2711, -50.9162) -> (77.0882, -50.8156)
  line L196 (77.0882, -50.8156) -> (76.903, -50.7194)
  line L197 (76.903, -50.7194) -> (76.7154, -50.6277)
  line L198 (76.7154, -50.6277) -> (76.8914, -50.2563)
  line L199 (76.8914, -50.2563) -> (76.9176, -50.1858)
  line L200 (76.9176, -50.1858) -> (76.9389, -50.113)
  line L201 (76.9389, -50.113) -> (76.9569, -50.0387)
  line L202 (76.9569, -50.0387) -> (76.9722, -49.9632)
  line L203 (76.9722, -49.9632) -> (76.9851, -49.8865)
  line L204 (76.9851, -49.8865) -> (76.9958, -49.8089)
  line L205 (76.9958, -49.8089) -> (77.0044, -49.7304)
  line L206 (77.0044, -49.7304) -> (77.0111, -49.6511)
  line L207 (77.0111, -49.6511) -> (77.0159, -49.5711)
  line L208 (77.0159, -49.5711) -> (77.0189, -49.4903)
  line L209 (77.0189, -49.4903) -> (77.0202, -49.4089)
  line L210 (77.0202, -49.4089) -> (77.0198, -49.3268)
  line L211 (77.0198, -49.3268) -> (76.8906, -49.2712)
  line L212 (76.8906, -49.2712) -> (76.7607, -49.2173)
  line L213 (76.7607, -49.2173) -> (76.6299, -49.1653)
  line L214 (76.6299, -49.1653) -> (76.5716, -49.2231)
  line L215 (76.5716, -49.2231) -> (76.515, -49.2816)
  line L216 (76.515, -49.2816) -> (76.46, -49.3408)
  line L217 (76.46, -49.3408) -> (76.4068, -49.4008)
  line L218 (76.4068, -49.4008) -> (76.3554, -49.4616)
  line L219 (76.3554, -49.4616) -> (76.306, -49.5232)
  line L220 (76.306, -49.5232) -> (76.2587, -49.5856)
  line L221 (76.2587, -49.5856) -> (76.2137, -49.6489)
  line L222 (76.2137, -49.6489) -> (76.171, -49.7132)
  line L223 (76.171, -49.7132) -> (76.1312, -49.7785)
  line L224 (76.1312, -49.7785) -> (76.0948, -49.845)
  line L225 (76.0948, -49.845) -> (76.0636, -49.9134)
  line L226 (76.0636, -49.9134) -> (75.9253, -50.3005)
  line L227 (75.9253, -50.3005) -> (75.7279, -50.2327)
  line L228 (75.7279, -50.2327) -> (75.5289, -50.1696)
  line L229 (75.5289, -50.1696) -> (75.3284, -50.1115)
  line L230 (75.3284, -50.1115) -> (75.1266, -50.0582)
  line L231 (75.1266, -50.0582) -> (75.2267, -49.6595)
  line L232 (75.2267, -49.6595) -> (75.2387, -49.5853)
  line L233 (75.2387, -49.5853) -> (75.2453, -49.5097)
  line L234 (75.2453, -49.5097) -> (75.2485, -49.4333)
  line L235 (75.2485, -49.4333) -> (75.2488, -49.3563)
  line L236 (75.2488, -49.3563) -> (75.2465, -49.2786)
  line L237 (75.2465, -49.2786) -> (75.2418, -49.2004)
  line L238 (75.2418, -49.2004) -> (75.235, -49.1217)
  line L239 (75.235, -49.1217) -> (75.226, -49.0427)
  line L240 (75.226, -49.0427) -> (75.2151, -48.9632)
  line L241 (75.2151, -48.9632) -> (75.2024, -48.8834)
  line L242 (75.2024, -48.8834) -> (75.1877, -48.8033)
  line L243 (75.1877, -48.8033) -> (75.1713, -48.7229)
  line L244 (75.1713, -48.7229) -> (75.0338, -48.6935)
  line L245 (75.0338, -48.6935) -> (74.8958, -48.666)
  line L246 (74.8958, -48.666) -> (74.7574, -48.6405)
  line L247 (74.7574, -48.6405) -> (74.7115, -48.7086)
  line L248 (74.7115, -48.7086) -> (74.6673, -48.777)
  line L249 (74.6673, -48.777) -> (74.625, -48.8458)
  line L250 (74.625, -48.8458) -> (74.5845, -48.9151)
  line L251 (74.5845, -48.9151) -> (74.546, -48.9847)
  line L252 (74.546, -48.9847) -> (74.5096, -49.0547)
  line L253 (74.5096, -49.0547) -> (74.4753, -49.1252)
  line L254 (74.4753, -49.1252) -> (74.4435, -49.1961)
  line L255 (74.4435, -49.1961) -> (74.4142, -49.2674)
  line L256 (74.4142, -49.2674) -> (74.3879, -49.3392)
  line L257 (74.3879, -49.3392) -> (74.3652, -49.4115)
  line L258 (74.3652, -49.4115) -> (74.3479, -49.4847)
  line L259 (74.3479, -49.4847) -> (74.2878, -49.8913)
  line L260 (74.2878, -49.8913) -> (74.0809, -49.8633)
  line L261 (74.0809, -49.8633) -> (73.8734, -49.8404)
  line L262 (73.8734, -49.8404) -> (73.6655, -49.8224)
  line L263 (73.6655, -49.8224) -> (73.4571, -49.8095)
  line L264 (73.4571, -49.8095) -> (73.4775, -49.399)
  line L265 (73.4775, -49.399) -> (73.4748, -49.3238)
  line L266 (73.4748, -49.3238) -> (73.4666, -49.2484)
  line L267 (73.4666, -49.2484) -> (73.4548, -49.1729)
  line L268 (73.4548, -49.1729) -> (73.4401, -49.0972)
  line L269 (73.4401, -49.0972) -> (73.4226, -49.0215)
  line L270 (73.4226, -49.0215) -> (73.4028, -48.9457)
  line L271 (73.4028, -48.9457) -> (73.3807, -48.8699)
  line L272 (73.3807, -48.8699) -> (73.3566, -48.7941)
  line L273 (73.3566, -48.7941) -> (73.3304, -48.7183)
  line L274 (73.3304, -48.7183) -> (73.3023, -48.6425)
  line L275 (73.3023, -48.6425) -> (73.2723, -48.5668)
  line L276 (73.2723, -48.5668) -> (73.2405, -48.4911)
  line L277 (73.2405, -48.4911) -> (73.0999, -48.4891)
  line L278 (73.0999, -48.4891) -> (72.9592, -48.4891)
  line L279 (72.9592, -48.4891) -> (72.8185, -48.4911)
  line L280 (72.8185, -48.4911) -> (72.7867, -48.5668)
  line L281 (72.7867, -48.5668) -> (72.7568, -48.6425)
  line L282 (72.7568, -48.6425) -> (72.7287, -48.7183)
  line L283 (72.7287, -48.7183) -> (72.7025, -48.7941)
  line L284 (72.7025, -48.7941) -> (72.6783, -48.8699)
  line L285 (72.6783, -48.8699) -> (72.6562, -48.9457)
  line L286 (72.6562, -48.9457) -> (72.6364, -49.0215)
  line L287 (72.6364, -49.0215) -> (72.619, -49.0972)
  line L288 (72.619, -49.0972) -> (72.6042, -49.1729)
  line L289 (72.6042, -49.1729) -> (72.5924, -49.2484)
  line L290 (72.5924, -49.2484) -> (72.5842, -49.3238)
  line L291 (72.5842, -49.3238) -> (72.5815, -49.399)
  line L292 (72.5815, -49.399) -> (72.6019, -49.8095)
  line L293 (72.6019, -49.8095) -> (72.3936, -49.8224)
  line L294 (72.3936, -49.8224) -> (72.1856, -49.8404)
  line L295 (72.1856, -49.8404) -> (71.9781, -49.8633)
  line L296 (71.9781, -49.8633) -> (71.7713, -49.8913)
  line L297 (71.7713, -49.8913) -> (71.7112, -49.4847)
  line L298 (71.7112, -49.4847) -> (71.6938, -49.4115)
  line L299 (71.6938, -49.4115) -> (71.6711, -49.3392)
  line L300 (71.6711, -49.3392) -> (71.6448, -49.2674)
  line L301 (71.6448, -49.2674) -> (71.6156, -49.1961)
  line L302 (71.6156, -49.1961) -> (71.5837, -49.1252)
  line L303 (71.5837, -49.1252) -> (71.5495, -49.0547)
  line L304 (71.5495, -49.0547) -> (71.513, -48.9847)
  line L305 (71.513, -48.9847) -> (71.4745, -48.9151)
  line L306 (71.4745, -48.9151) -> (71.4341, -48.8458)
  line L307 (71.4341, -48.8458) -> (71.3917, -48.777)
  line L308 (71.3917, -48.777) -> (71.3475, -48.7086)
  line L309 (71.3475, -48.7086) -> (71.3016, -48.6405)
  line L310 (71.3016, -48.6405) -> (71.1633, -48.666)
  line L311 (71.1633, -48.666) -> (71.0253, -48.6935)
  line L312 (71.0253, -48.6935) -> (70.8877, -48.7229)
  line L313 (70.8877, -48.7229) -> (70.8713, -48.8033)
  line L314 (70.8713, -48.8033) -> (70.8567, -48.8834)
  line L315 (70.8567, -48.8834) -> (70.8439, -48.9632)
  line L316 (70.8439, -48.9632) -> (70.833, -49.0427)
  line L317 (70.833, -49.0427) -> (70.8241, -49.1217)
  line L318 (70.8241, -49.1217) -> (70.8172, -49.2004)
  line L319 (70.8172, -49.2004) -> (70.8126, -49.2786)
  line L320 (70.8126, -49.2786) -> (70.8103, -49.3563)
  line L321 (70.8103, -49.3563) -> (70.8105, -49.4333)
  line L322 (70.8105, -49.4333) -> (70.8137, -49.5097)
  line L323 (70.8137, -49.5097) -> (70.8204, -49.5853)
  line L324 (70.8204, -49.5853) -> (70.8324, -49.6595)
  line L325 (70.8324, -49.6595) -> (70.9325, -50.0582)
  line L326 (70.9325, -50.0582) -> (70.7306, -50.1115)
  line L327 (70.7306, -50.1115) -> (70.5302, -50.1696)
  line L328 (70.5302, -50.1696) -> (70.3312, -50.2327)
  line L329 (70.3312, -50.2327) -> (70.1337, -50.3005)
  line L330 (70.1337, -50.3005) -> (69.9955, -49.9134)
  line L331 (69.9955, -49.9134) -> (69.9642, -49.845)
  line L332 (69.9642, -49.845) -> (69.9278, -49.7785)
  line L333 (69.9278, -49.7785) -> (69.888, -49.7132)
  line L334 (69.888, -49.7132) -> (69.8454, -49.6489)
  line L335 (69.8454, -49.6489) -> (69.8003, -49.5856)
  line L336 (69.8003, -49.5856) -> (69.753, -49.5232)
  line L337 (69.753, -49.5232) -> (69.7036, -49.4616)
  line L338 (69.7036, -49.4616) -> (69.6523, -49.4008)
  line L339 (69.6523, -49.4008) -> (69.5991, -49.3408)
  line L340 (69.5991, -49.3408) -> (69.5441, -49.2816)
  line L341 (69.5441, -49.2816) -> (69.4874, -49.2231)
  line L342 (69.4874, -49.2231) -> (69.4291, -49.1653)
  line L343 (69.4291, -49.1653) -> (69.2984, -49.2173)
  line L344 (69.2984, -49.2173) -> (69.1684, -49.2712)
  line L345 (69.1684, -49.2712) -> (69.0392, -49.3268)
  line L346 (69.0392, -49.3268) -> (69.0388, -49.4089)
  line L347 (69.0388, -49.4089) -> (69.0401, -49.4903)
  line L348 (69.0401, -49.4903) -> (69.0431, -49.5711)
  line L349 (69.0431, -49.5711) -> (69.0479, -49.6511)
  line L350 (69.0479, -49.6511) -> (69.0546, -49.7304)
  line L351 (69.0546, -49.7304) -> (69.0633, -49.8089)
  line L352 (69.0633, -49.8089) -> (69.0739, -49.8865)
  line L353 (69.0739, -49.8865) -> (69.0868, -49.9632)
  line L354 (69.0868, -49.9632) -> (69.1021, -50.0387)
  line L355 (69.1021, -50.0387) -> (69.1201, -50.113)
  line L356 (69.1201, -50.113) -> (69.1414, -50.1858)
  line L357 (69.1414, -50.1858) -> (69.1677, -50.2563)
  line L358 (69.1677, -50.2563) -> (69.3436, -50.6277)
  line L359 (69.3436, -50.6277) -> (69.1561, -50.7194)
  line L360 (69.1561, -50.7194) -> (68.9708, -50.8156)
  line L361 (68.9708, -50.8156) -> (68.7879, -50.9162)
  line L362 (68.7879, -50.9162) -> (68.6075, -51.0212)
  line L363 (68.6075, -51.0212) -> (68.3964, -50.6685)
  line L364 (68.3964, -50.6685) -> (68.3524, -50.6076)
  line L365 (68.3524, -50.6076) -> (68.3037, -50.5494)
  line L366 (68.3037, -50.5494) -> (68.2519, -50.4932)
  line L367 (68.2519, -50.4932) -> (68.1976, -50.4385)
  line L368 (68.1976, -50.4385) -> (68.141, -50.3852)
  line L369 (68.141, -50.3852) -> (68.0824, -50.3332)
  line L370 (68.0824, -50.3332) -> (68.022, -50.2824)
  line L371 (68.022, -50.2824) -> (67.9598, -50.2328)
  line L372 (67.9598, -50.2328) -> (67.8959, -50.1843)
  line L373 (67.8959, -50.1843) -> (67.8304, -50.1369)
  line L374 (67.8304, -50.1369) -> (67.7634, -50.0906)
  line L375 (67.7634, -50.0906) -> (67.695, -50.0454)
  line L376 (67.695, -50.0454) -> (67.5769, -50.1219)
  line L377 (67.5769, -50.1219) -> (67.4599, -50.2)
  line L378 (67.4599, -50.2) -> (67.3441, -50.2798)
  line L379 (67.3441, -50.2798) -> (67.3597, -50.3604)
  line L380 (67.3597, -50.3604) -> (67.3768, -50.44)
  line L381 (67.3768, -50.44) -> (67.3956, -50.5186)
  line L382 (67.3956, -50.5186) -> (67.4159, -50.5962)
  line L383 (67.4159, -50.5962) -> (67.4379, -50.6727)
  line L384 (67.4379, -50.6727) -> (67.4617, -50.748)
  line L385 (67.4617, -50.748) -> (67.4873, -50.822)
  line L386 (67.4873, -50.822) -> (67.5149, -50.8946)
  line L387 (67.5149, -50.8946) -> (67.5446, -50.9657)
  line L388 (67.5446, -50.9657) -> (67.5768, -51.0351)
  line L389 (67.5768, -51.0351) -> (67.6119, -51.1023)
  line L390 (67.6119, -51.1023) -> (67.6514, -51.1663)
  line L391 (67.6514, -51.1663) -> (67.8964, -51.4963)
  line L392 (67.8964, -51.4963) -> (67.7304, -51.6228)
  line L393 (67.7304, -51.6228) -> (67.5674, -51.7533)
  line L394 (67.5674, -51.7533) -> (67.4076, -51.8877)
  line L395 (67.4076, -51.8877) -> (67.2512, -52.0259)
  line L396 (67.2512, -52.0259) -> (66.9753, -51.7211)
  line L397 (66.9753, -51.7211) -> (66.9203, -51.6699)
  line L398 (66.9203, -51.6699) -> (66.8612, -51.6224)
  line L399 (66.8612, -51.6224) -> (66.7994, -51.5773)
  line L400 (66.7994, -51.5773) -> (66.7355, -51.5343)
  line L401 (66.7355, -51.5343) -> (66.6696, -51.493)
  line L402 (66.6696, -51.493) -> (66.602, -51.4535)
  line L403 (66.602, -51.4535) -> (66.5328, -51.4155)
  line L404 (66.5328, -51.4155) -> (66.4621, -51.379)
  line L405 (66.4621, -51.379) -> (66.39, -51.3439)
  line L406 (66.39, -51.3439) -> (66.3165, -51.3102)
  line L407 (66.3165, -51.3102) -> (66.2418, -51.2778)
  line L408 (66.2418, -51.2778) -> (66.1658, -51.2468)
  line L409 (66.1658, -51.2468) -> (66.0649, -51.3448)
  line L410 (66.0649, -51.3448) -> (65.9655, -51.4443)
  line L411 (65.9655, -51.4443) -> (65.8674, -51.5452)
  line L412 (65.8674, -51.5452) -> (65.8984, -51.6212)
  line L413 (65.8984, -51.6212) -> (65.9308, -51.6959)
  line L414 (65.9308, -51.6959) -> (65.9645, -51.7694)
  line L415 (65.9645, -51.7694) -> (65.9996, -51.8415)
  line L416 (65.9996, -51.8415) -> (66.0361, -51.9122)
  line L417 (66.0361, -51.9122) -> (66.0741, -51.9814)
  line L418 (66.0741, -51.9814) -> (66.1137, -52.049)
  line L419 (66.1137, -52.049) -> (66.1549, -52.1149)
  line L420 (66.1549, -52.1149) -> (66.1979, -52.1788)
  line L421 (66.1979, -52.1788) -> (66.243, -52.2406)
  line L422 (66.243, -52.2406) -> (66.2906, -52.2997)
  line L423 (66.2906, -52.2997) -> (66.3418, -52.3547)
  line L424 (66.3418, -52.3547) -> (66.6465, -52.6306)
  line L425 (66.6465, -52.6306) -> (66.5083, -52.787)
  line L426 (66.5083, -52.787) -> (66.3739, -52.9468)
  line L427 (66.3739, -52.9468) -> (66.2434, -53.1097)
  line L428 (66.2434, -53.1097) -> (66.117, -53.2758)
  line L429 (66.117, -53.2758) -> (65.787, -53.0307)
  line L430 (65.787, -53.0307) -> (65.723, -52.9913)
  line L431 (65.723, -52.9913) -> (65.6557, -52.9562)
  line L432 (65.6557, -52.9562) -> (65.5864, -52.924)
  line L433 (65.5864, -52.924) -> (65.5152, -52.8943)
  line L434 (65.5152, -52.8943) -> (65.4426, -52.8667)
  line L435 (65.4426, -52.8667) -> (65.3686, -52.8411)
  line L436 (65.3686, -52.8411) -> (65.2933, -52.8173)
  line L437 (65.2933, -52.8173) -> (65.2168, -52.7953)
  line L438 (65.2168, -52.7953) -> (65.1392, -52.7749)
  line L439 (65.1392, -52.7749) -> (65.0606, -52.7562)
  line L440 (65.0606, -52.7562) -> (64.981, -52.7391)
  line L441 (64.981, -52.7391) -> (64.9004, -52.7234)
  line L442 (64.9004, -52.7234) -> (64.8206, -52.8393)
  line L443 (64.8206, -52.8393) -> (64.7425, -52.9563)
  line L444 (64.7425, -52.9563) -> (64.666, -53.0743)
  line L445 (64.666, -53.0743) -> (64.7112, -53.1428)
  line L446 (64.7112, -53.1428) -> (64.7575, -53.2098)
  line L447 (64.7575, -53.2098) -> (64.8049, -53.2753)
  line L448 (64.8049, -53.2753) -> (64.8534, -53.3391)
  line L449 (64.8534, -53.3391) -> (64.903, -53.4014)
  line L450 (64.903, -53.4014) -> (64.9538, -53.4618)
  line L451 (64.9538, -53.4618) -> (65.0058, -53.5204)
  line L452 (65.0058, -53.5204) -> (65.0591, -53.577)
  line L453 (65.0591, -53.577) -> (65.1138, -53.6313)
  line L454 (65.1138, -53.6313) -> (65.17, -53.6831)
  line L455 (65.17, -53.6831) -> (65.2282, -53.7318)
  line L456 (65.2282, -53.7318) -> (65.2891, -53.7758)
  line L457 (65.2891, -53.7758) -> (65.6418, -53.9869)
  line L458 (65.6418, -53.9869) -> (65.5368, -54.1673)
  line L459 (65.5368, -54.1673) -> (65.4362, -54.3502)
  line L460 (65.4362, -54.3502) -> (65.34, -54.5355)
  line L461 (65.34, -54.5355) -> (65.2484, -54.723)
  line L462 (65.2484, -54.723) -> (64.8769, -54.547)
  line L463 (64.8769, -54.547) -> (64.8064, -54.5208)
  line L464 (64.8064, -54.5208) -> (64.7336, -54.4995)
  line L465 (64.7336, -54.4995) -> (64.6593, -54.4815)
  line L466 (64.6593, -54.4815) -> (64.5838, -54.4662)
  line L467 (64.5838, -54.4662) -> (64.5071, -54.4533)
  line L468 (64.5071, -54.4533) -> (64.4295, -54.4426)
  line L469 (64.4295, -54.4426) -> (64.3511, -54.434)
  line L470 (64.3511, -54.434) -> (64.2718, -54.4273)
  line L471 (64.2718, -54.4273) -> (64.1917, -54.4225)
  line L472 (64.1917, -54.4225) -> (64.111, -54.4195)
  line L473 (64.111, -54.4195) -> (64.0295, -54.4182)
  line L474 (64.0295, -54.4182) -> (63.9475, -54.4186)
  line L475 (63.9475, -54.4186) -> (63.8918, -54.5478)
  line L476 (63.8918, -54.5478) -> (63.8379, -54.6778)
  line L477 (63.8379, -54.6778) -> (63.786, -54.8085)
  line L478 (63.786, -54.8085) -> (63.8437, -54.8668)
  line L479 (63.8437, -54.8668) -> (63.9022, -54.9235)
  line L480 (63.9022, -54.9235) -> (63.9614, -54.9784)
  line L481 (63.9614, -54.9784) -> (64.0215, -55.0316)
  line L482 (64.0215, -55.0316) -> (64.0823, -55.083)
  line L483 (64.0823, -55.083) -> (64.1438, -55.1324)
  line L484 (64.1438, -55.1324) -> (64.2063, -55.1797)
  line L485 (64.2063, -55.1797) -> (64.2696, -55.2248)
  line L486 (64.2696, -55.2248) -> (64.3338, -55.2674)
  line L487 (64.3338, -55.2674) -> (64.3991, -55.3072)
  line L488 (64.3991, -55.3072) -> (64.4656, -55.3436)
  line L489 (64.4656, -55.3436) -> (64.534, -55.3749)
  line L490 (64.534, -55.3749) -> (64.9211, -55.5131)
  line L491 (64.9211, -55.5131) -> (64.8533, -55.7105)
  line L492 (64.8533, -55.7105) -> (64.7903, -55.9095)
  line L493 (64.7903, -55.9095) -> (64.7321, -56.11)
  line L494 (64.7321, -56.11) -> (64.6788, -56.3119)
  line L495 (64.6788, -56.3119) -> (64.2801, -56.2117)
  line L496 (64.2801, -56.2117) -> (64.2059, -56.1998)
  line L497 (64.2059, -56.1998) -> (64.1304, -56.1931)
  line L498 (64.1304, -56.1931) -> (64.054, -56.1899)
  line L499 (64.054, -56.1899) -> (63.9769, -56.1896)
  line L500 (63.9769, -56.1896) -> (63.8992, -56.192)
  line L501 (63.8992, -56.192) -> (63.821, -56.1966)
  line L502 (63.821, -56.1966) -> (63.7424, -56.2035)
  line L503 (63.7424, -56.2035) -> (63.6633, -56.2124)
  line L504 (63.6633, -56.2124) -> (63.5838, -56.2233)
  line L505 (63.5838, -56.2233) -> (63.504, -56.2361)